Autodesk Fusion 360 part; units mm, degrees
(part 34 of 40)
  line L8870 (236.8217, 91.8506) -> (236.8425, 91.6948) construction
  line L8871 (236.8425, 91.6948) -> (236.8621, 91.5386) construction
  line L8872 (236.8621, 91.5386) -> (236.8805, 91.3821) construction
  line L8873 (236.8805, 91.3821) -> (236.8978, 91.2253) construction
  line L8874 (236.8978, 91.2253) -> (236.9138, 91.0682) construction
  line L8875 (236.9138, 91.0682) -> (236.9285, 90.9107) construction
  line L8876 (236.9285, 90.9107) -> (236.9418, 90.7529) construction
  line L8877 (236.9418, 90.7529) -> (236.9538, 90.5947) construction
  line L8878 (236.9538, 90.5947) -> (236.9645, 90.4362) construction
  line L8879 (236.9645, 90.4362) -> (236.974, 90.2774) construction
  line L8880 (236.974, 90.2774) -> (236.9824, 90.1183) construction
  line L8881 (236.9824, 90.1183) -> (236.9897, 89.9589) construction
  line L8882 (236.9897, 89.9589) -> (236.9958, 89.7993) construction
  line L8883 (236.9958, 89.7993) -> (237.0009, 89.6395) construction
  line L8884 (237.0009, 89.6395) -> (237.0049, 89.4794) construction
  line L8885 (237.0049, 89.4794) -> (237.0077, 89.3191) construction
  line L8886 (237.0077, 89.3191) -> (237.0096, 89.1585) construction
  line L8887 (237.0096, 89.1585) -> (237.0103, 88.9977) construction
  line L8888 (237.0103, 88.9977) -> (237.01, 88.8367) construction
  line L8889 (237.01, 88.8367) -> (237.0086, 88.6755) construction
  line L8890 (237.0086, 88.6755) -> (237.0062, 88.5141) construction
  line L8891 (237.0062, 88.5141) -> (237.0028, 88.3525) construction
  line L8892 (237.0028, 88.3525) -> (236.9985, 88.1907) construction
  line L8893 (236.9985, 88.1907) -> (236.9931, 88.0288) construction
  line L8894 (236.9931, 88.0288) -> (236.9868, 87.8666) construction
  line L8895 (236.9868, 87.8666) -> (236.9795, 87.7043) construction
  line L8896 (236.9795, 87.7043) -> (236.9712, 87.5419) construction
  line L8897 (236.9712, 87.5419) -> (236.962, 87.3793) construction
  line L8898 (236.962, 87.3793) -> (236.9519, 87.2165) construction
  line L8899 (236.9519, 87.2165) -> (236.9408, 87.0536) construction
  line L8900 (236.9408, 87.0536) -> (236.9287, 86.8905) construction
  line L8901 (236.9287, 86.8905) -> (236.9158, 86.7273) construction
  line L8902 (236.9158, 86.7273) -> (236.902, 86.564) construction
  line L8903 (236.902, 86.564) -> (236.8872, 86.4005) construction
  line L8904 (236.8872, 86.4005) -> (236.8716, 86.2369) construction
  line L8905 (236.8716, 86.2369) -> (236.855, 86.0732) construction
  line L8906 (236.855, 86.0732) -> (236.8376, 85.9094) construction
  line L8907 (236.8376, 85.9094) -> (236.8193, 85.7455) construction
  line L8908 (236.8193, 85.7455) -> (236.8001, 85.5815) construction
  line L8909 (236.8001, 85.5815) -> (236.78, 85.4174) construction
  line L8910 (236.78, 85.4174) -> (236.7591, 85.2532) construction
  line L8911 (236.7591, 85.2532) -> (236.7374, 85.0889) construction
  line L8912 (236.7374, 85.0889) -> (236.7148, 84.9245) construction
  line L8913 (236.7148, 84.9245) -> (236.6913, 84.76) construction
  line L8914 (236.6913, 84.76) -> (236.667, 84.5954) construction
  line L8915 (236.667, 84.5954) -> (236.6418, 84.4308) construction
  line L8916 (236.6418, 84.4308) -> (236.6159, 84.266) construction
  line L8917 (236.6159, 84.266) -> (236.5891, 84.1013) construction
  line L8918 (236.5891, 84.1013) -> (236.5614, 83.9364) construction
  line L8919 (236.5614, 83.9364) -> (236.533, 83.7715) construction
  line L8920 (236.533, 83.7715) -> (236.5038, 83.6065) construction
  line L8921 (236.5038, 83.6065) -> (236.4737, 83.4415) construction
  line L8922 (236.4737, 83.4415) -> (236.4428, 83.2764) construction
  line L8923 (236.4428, 83.2764) -> (236.4112, 83.1113) construction
  line L8924 (236.4112, 83.1113) -> (236.3852, 82.9792) construction
  line L8925 (236.3852, 82.9792) -> (236.3654, 82.8801) construction
  line L8926 (236.3654, 82.8801) -> (236.352, 82.814) construction
  line L8927 (236.352, 82.814) -> (236.3452, 82.7809) construction
  arc A219 (171.9828, 209.0993) -> (168.332, 206.4469) centre (212.132, 150) ccw
  arc A220 (181.8522, 201.1066) -> (184.5338, 200.3721) centre (183.5728, 202.1261) ccw
  arc A221 (204.8514, 206.9737) -> (206.5892, 209.1442) centre (204.5979, 208.9575) ccw
  spline S119 degree 5 poles (206.4369, 89.2315) (206.4341, 89.2007) (206.4291, 89.1391) (206.4242, 89.0467) (206.4223, 88.9234) (206.4264, 88.769) (206.4351, 88.6144) (206.4466, 88.4597) (206.4597, 88.305) (206.4737, 88.1502) (206.4889, 87.9955) (206.5055, 87.8407) (206.524, 87.686) (206.5449, 87.5312) (206.5679, 87.3765) (206.593, 87.2218) (206.6199, 87.0671) (206.6482, 86.9125) (206.6778, 86.7579) (206.7087, 86.6034) (206.7407, 86.4489) (206.7741, 86.2945) (206.8088, 86.1402) (206.8449, 85.986) (206.8823, 85.8318) (206.9211, 85.6778) (206.9611, 85.5238) (207.0023, 85.3699) (207.0447, 85.2161) (207.0881, 85.0624) (207.1327, 84.9088) (207.1784, 84.7553) (207.2252, 84.602) (207.2731, 84.4487) (207.3221, 84.2956) (207.3721, 84.1426) (207.4233, 83.9897) (207.4754, 83.8369) (207.5285, 83.6842) (207.5827, 83.5317) (207.6378, 83.3794) (207.694, 83.2271) (207.751, 83.075) (207.8091, 82.923) (207.8681, 82.7712) (207.9281, 82.6196) (207.989, 82.468) (208.0508, 82.3167) (208.1135, 82.1655) (208.1772, 82.0144) (208.2417, 81.8635) (208.3071, 81.7128) (208.3735, 81.5622) (208.4407, 81.4118) (208.5087, 81.2616) (208.5777, 81.1115) (208.6474, 80.9616) (208.7181, 80.8119) (208.7895, 80.6624) (208.8619, 80.513) (208.935, 80.3638) (209.009, 80.2148) (209.0838, 80.066) (209.1594, 79.9174) (209.2358, 79.7689) (209.313, 79.6207) (209.391, 79.4726) (209.4698, 79.3248) (209.5494, 79.1771) (209.6297, 79.0297) (209.7109, 78.8824) (209.7764, 78.7648) (209.8259, 78.6766) (209.8591, 78.6179) (209.8757, 78.5885) knots 0 0 0 0 0 0 0.01428571 0.02857143 0.04285714 0.05714286 0.07142857 0.08571429 0.1 0.11428571 0.12857143 0.14285714 0.15714286 0.17142857 0.18571429 0.2 0.21428571 0.22857143 0.24285714 0.25714286 0.27142857 0.28571429 0.3 0.31428571 0.32857143 0.34285714 0.35714286 0.37142857 0.38571429 0.4 0.41428571 0.42857143 0.44285714 0.45714286 0.47142857 0.48571429 0.5 0.51428571 0.52857143 0.54285714 0.55714286 0.57142857 0.58571429 0.6 0.61428571 0.62857143 0.64285714 0.65714286 0.67142857 0.68571429 0.7 0.71428571 0.72857143 0.74285714 0.75714286 0.77142857 0.78571429 0.8 0.81428571 0.82857143 0.84285714 0.85714286 0.87142857 0.88571429 0.9 0.91428571 0.92857143 0.94285714 0.95714286 0.97142857 0.98571429 1 1 1 1 1 1
  line L8928 (206.4369, 89.2315) -> (206.4341, 89.2007) construction
  line L8929 (206.4341, 89.2007) -> (206.4291, 89.1391) construction
  line L8930 (206.4291, 89.1391) -> (206.4242, 89.0467) construction
  line L8931 (206.4242, 89.0467) -> (206.4223, 88.9234) construction
  line L8932 (206.4223, 88.9234) -> (206.4264, 88.769) construction
  line L8933 (206.4264, 88.769) -> (206.4351, 88.6144) construction
  line L8934 (206.4351, 88.6144) -> (206.4466, 88.4597) construction
  line L8935 (206.4466, 88.4597) -> (206.4597, 88.305) construction
  line L8936 (206.4597, 88.305) -> (206.4737, 88.1502) construction
  line L8937 (206.4737, 88.1502) -> (206.4889, 87.9955) construction
  line L8938 (206.4889, 87.9955) -> (206.5055, 87.8407) construction
  line L8939 (206.5055, 87.8407) -> (206.524, 87.686) construction
  line L8940 (206.524, 87.686) -> (206.5449, 87.5312) construction
  line L8941 (206.5449, 87.5312) -> (206.5679, 87.3765) construction
  line L8942 (206.5679, 87.3765) -> (206.593, 87.2218) construction
  line L8943 (206.593, 87.2218) -> (206.6199, 87.0671) construction
  line L8944 (206.6199, 87.0671) -> (206.6482, 86.9125) construction
  line L8945 (206.6482, 86.9125) -> (206.6778, 86.7579) construction
  line L8946 (206.6778, 86.7579) -> (206.7087, 86.6034) construction
  line L8947 (206.7087, 86.6034) -> (206.7407, 86.4489) construction
  line L8948 (206.7407, 86.4489) -> (206.7741, 86.2945) construction
  line L8949 (206.7741, 86.2945) -> (206.8088, 86.1402) construction
  line L8950 (206.8088, 86.1402) -> (206.8449, 85.986) construction
  line L8951 (206.8449, 85.986) -> (206.8823, 85.8318) construction
  line L8952 (206.8823, 85.8318) -> (206.9211, 85.6778) construction
  line L8953 (206.9211, 85.6778) -> (206.9611, 85.5238) construction
  line L8954 (206.9611, 85.5238) -> (207.0023, 85.3699) construction
  line L8955 (207.0023, 85.3699) -> (207.0447, 85.2161) construction
  line L8956 (207.0447, 85.2161) -> (207.0881, 85.0624) construction
  line L8957 (207.0881, 85.0624) -> (207.1327, 84.9088) construction
  line L8958 (207.1327, 84.9088) -> (207.1784, 84.7553) construction
  line L8959 (207.1784, 84.7553) -> (207.2252, 84.602) construction
  line L8960 (207.2252, 84.602) -> (207.2731, 84.4487) construction
  line L8961 (207.2731, 84.4487) -> (207.3221, 84.2956) construction
  line L8962 (207.3221, 84.2956) -> (207.3721, 84.1426) construction
  line L8963 (207.3721, 84.1426) -> (207.4233, 83.9897) construction
  line L8964 (207.4233, 83.9897) -> (207.4754, 83.8369) construction
  line L8965 (207.4754, 83.8369) -> (207.5285, 83.6842) construction
  line L8966 (207.5285, 83.6842) -> (207.5827, 83.5317) construction
  line L8967 (207.5827, 83.5317) -> (207.6378, 83.3794) construction
  line L8968 (207.6378, 83.3794) -> (207.694, 83.2271) construction
  line L8969 (207.694, 83.2271) -> (207.751, 83.075) construction
  line L8970 (207.751, 83.075) -> (207.8091, 82.923) construction
  line L8971 (207.8091, 82.923) -> (207.8681, 82.7712) construction
  line L8972 (207.8681, 82.7712) -> (207.9281, 82.6196) construction
  line L8973 (207.9281, 82.6196) -> (207.989, 82.468) construction
  line L8974 (207.989, 82.468) -> (208.0508, 82.3167) construction
  line L8975 (208.0508, 82.3167) -> (208.1135, 82.1655) construction
  line L8976 (208.1135, 82.1655) -> (208.1772, 82.0144) construction
  line L8977 (208.1772, 82.0144) -> (208.2417, 81.8635) construction
  line L8978 (208.2417, 81.8635) -> (208.3071, 81.7128) construction
  line L8979 (208.3071, 81.7128) -> (208.3735, 81.5622) construction
  line L8980 (208.3735, 81.5622) -> (208.4407, 81.4118) construction
  line L8981 (208.4407, 81.4118) -> (208.5087, 81.2616) construction
  line L8982 (208.5087, 81.2616) -> (208.5777, 81.1115) construction
  line L8983 (208.5777, 81.1115) -> (208.6474, 80.9616) construction
  line L8984 (208.6474, 80.9616) -> (208.7181, 80.8119) construction
  line L8985 (208.7181, 80.8119) -> (208.7895, 80.6624) construction
  line L8986 (208.7895, 80.6624) -> (208.8619, 80.513) construction
  line L8987 (208.8619, 80.513) -> (208.935, 80.3638) construction
  line L8988 (208.935, 80.3638) -> (209.009, 80.2148) construction
  line L8989 (209.009, 80.2148) -> (209.0838, 80.066) construction
  line L8990 (209.0838, 80.066) -> (209.1594, 79.9174) construction
  line L8991 (209.1594, 79.9174) -> (209.2358, 79.7689) construction
  line L8992 (209.2358, 79.7689) -> (209.313, 79.6207) construction
  line L8993 (209.313, 79.6207) -> (209.391, 79.4726) construction
  line L8994 (209.391, 79.4726) -> (209.4698, 79.3248) construction
  line L8995 (209.4698, 79.3248) -> (209.5494, 79.1771) construction
  line L8996 (209.5494, 79.1771) -> (209.6297, 79.0297) construction
  line L8997 (209.6297, 79.0297) -> (209.7109, 78.8824) construction
  line L8998 (209.7109, 78.8824) -> (209.7764, 78.7648) construction
  line L8999 (209.7764, 78.7648) -> (209.8259, 78.6766) construction
  line L9000 (209.8259, 78.6766) -> (209.8591, 78.6179) construction
  line L9001 (209.8591, 78.6179) -> (209.8757, 78.5885) construction
  arc A222 (279.3511, 125.7868) -> (280.7456, 130.0785) centre (212.132, 150) ccw
  arc A223 (280.7456, 169.9215) -> (279.3511, 174.2132) centre (212.132, 150) ccw
  arc A224 (209.8757, 78.5885) -> (214.3883, 78.5885) centre (212.132, 150) ccw
  arc A225 (283.5435, 147.7437) -> (283.5435, 152.2563) centre (212.132, 150) ccw
  spline S120 degree 5 poles (206.4369, 210.7685) (206.4341, 210.7993) (206.4291, 210.8609) (206.4242, 210.9533) (206.4223, 211.0766) (206.4264, 211.231) (206.4351, 211.3856) (206.4466, 211.5403) (206.4597, 211.695) (206.4737, 211.8498) (206.4889, 212.0045) (206.5055, 212.1593) (206.524, 212.314) (206.5449, 212.4688) (206.5679, 212.6235) (206.593, 212.7782) (206.6199, 212.9329) (206.6482, 213.0875) (206.6778, 213.2421) (206.7087, 213.3966) (206.7407, 213.5511) (206.7741, 213.7055) (206.8088, 213.8598) (206.8449, 214.014) (206.8823, 214.1682) (206.9211, 214.3222) (206.9611, 214.4762) (207.0023, 214.6301) (207.0447, 214.7839) (207.0881, 214.9376) (207.1327, 215.0912) (207.1784, 215.2447) (207.2252, 215.398) (207.2731, 215.5513) (207.3221, 215.7044) (207.3721, 215.8574) (207.4233, 216.0103) (207.4754, 216.1631) (207.5285, 216.3158) (207.5827, 216.4683) (207.6378, 216.6206) (207.694, 216.7729) (207.751, 216.925) (207.8091, 217.077) (207.8681, 217.2288) (207.9281, 217.3804) (207.989, 217.532) (208.0508, 217.6833) (208.1135, 217.8345) (208.1772, 217.9856) (208.2417, 218.1365) (208.3071, 218.2872) (208.3735, 218.4378) (208.4407, 218.5882) (208.5087, 218.7384) (208.5777, 218.8885) (208.6474, 219.0384) (208.7181, 219.1881) (208.7895, 219.3376) (208.8619, 219.487) (208.935, 219.6362) (209.009, 219.7852) (209.0838, 219.934) (209.1594, 220.0826) (209.2358, 220.2311) (209.313, 220.3793) (209.391, 220.5274) (209.4698, 220.6752) (209.5494, 220.8229) (209.6297, 220.9703) (209.7109, 221.1176) (209.7764, 221.2352) (209.8259, 221.3234) (209.8591, 221.3821) (209.8757, 221.4115) knots 0 0 0 0 0 0 0.01428571 0.02857143 0.04285714 0.05714286 0.07142857 0.08571429 0.1 0.11428571 0.12857143 0.14285714 0.15714286 0.17142857 0.18571429 0.2 0.21428571 0.22857143 0.24285714 0.25714286 0.27142857 0.28571429 0.3 0.31428571 0.32857143 0.34285714 0.35714286 0.37142857 0.38571429 0.4 0.41428571 0.42857143 0.44285714 0.45714286 0.47142857 0.48571429 0.5 0.51428571 0.52857143 0.54285714 0.55714286 0.57142857 0.58571429 0.6 0.61428571 0.62857143 0.64285714 0.65714286 0.67142857 0.68571429 0.7 0.71428571 0.72857143 0.74285714 0.75714286 0.77142857 0.78571429 0.8 0.81428571 0.82857143 0.84285714 0.85714286 0.87142857 0.88571429 0.9 0.91428571 0.92857143 0.94285714 0.95714286 0.97142857 0.98571429 1 1 1 1 1 1
  line L9002 (206.4369, 210.7685) -> (206.4341, 210.7993) construction
  line L9003 (206.4341, 210.7993) -> (206.4291, 210.8609) construction
  line L9004 (206.4291, 210.8609) -> (206.4242, 210.9533) construction
  line L9005 (206.4242, 210.9533) -> (206.4223, 211.0766) construction
  line L9006 (206.4223, 211.0766) -> (206.4264, 211.231) construction
  line L9007 (206.4264, 211.231) -> (206.4351, 211.3856) construction
  line L9008 (206.4351, 211.3856) -> (206.4466, 211.5403) construction
  line L9009 (206.4466, 211.5403) -> (206.4597, 211.695) construction
  line L9010 (206.4597, 211.695) -> (206.4737, 211.8498) construction
  line L9011 (206.4737, 211.8498) -> (206.4889, 212.0045) construction
  line L9012 (206.4889, 212.0045) -> (206.5055, 212.1593) construction
  line L9013 (206.5055, 212.1593) -> (206.524, 212.314) construction
  line L9014 (206.524, 212.314) -> (206.5449, 212.4688) construction
  line L9015 (206.5449, 212.4688) -> (206.5679, 212.6235) construction
  line L9016 (206.5679, 212.6235) -> (206.593, 212.7782) construction
  line L9017 (206.593, 212.7782) -> (206.6199, 212.9329) construction
  line L9018 (206.6199, 212.9329) -> (206.6482, 213.0875) construction
  line L9019 (206.6482, 213.0875) -> (206.6778, 213.2421) construction
  line L9020 (206.6778, 213.2421) -> (206.7087, 213.3966) construction
  line L9021 (206.7087, 213.3966) -> (206.7407, 213.5511) construction
  line L9022 (206.7407, 213.5511) -> (206.7741, 213.7055) construction
  line L9023 (206.7741, 213.7055) -> (206.8088, 213.8598) construction
  line L9024 (206.8088, 213.8598) -> (206.8449, 214.014) construction
  line L9025 (206.8449, 214.014) -> (206.8823, 214.1682) construction
  line L9026 (206.8823, 214.1682) -> (206.9211, 214.3222) construction
  line L9027 (206.9211, 214.3222) -> (206.9611, 214.4762) construction
  line L9028 (206.9611, 214.4762) -> (207.0023, 214.6301) construction
  line L9029 (207.0023, 214.6301) -> (207.0447, 214.7839) construction
  line L9030 (207.0447, 214.7839) -> (207.0881, 214.9376) construction
  line L9031 (207.0881, 214.9376) -> (207.1327, 215.0912) construction
  line L9032 (207.1327, 215.0912) -> (207.1784, 215.2447) construction
  line L9033 (207.1784, 215.2447) -> (207.2252, 215.398) construction
  line L9034 (207.2252, 215.398) -> (207.2731, 215.5513) construction
  line L9035 (207.2731, 215.5513) -> (207.3221, 215.7044) construction
  line L9036 (207.3221, 215.7044) -> (207.3721, 215.8574) construction
  line L9037 (207.3721, 215.8574) -> (207.4233, 216.0103) construction
  line L9038 (207.4233, 216.0103) -> (207.4754, 216.1631) construction
  line L9039 (207.4754, 216.1631) -> (207.5285, 216.3158) construction
  line L9040 (207.5285, 216.3158) -> (207.5827, 216.4683) construction
  line L9041 (207.5827, 216.4683) -> (207.6378, 216.6206) construction
  line L9042 (207.6378, 216.6206) -> (207.694, 216.7729) construction
  line L9043 (207.694, 216.7729) -> (207.751, 216.925) construction
  line L9044 (207.751, 216.925) -> (207.8091, 217.077) construction
  line L9045 (207.8091, 217.077) -> (207.8681, 217.2288) construction
  line L9046 (207.8681, 217.2288) -> (207.9281, 217.3804) construction
  line L9047 (207.9281, 217.3804) -> (207.989, 217.532) construction
  line L9048 (207.989, 217.532) -> (208.0508, 217.6833) construction
  line L9049 (208.0508, 217.6833) -> (208.1135, 217.8345) construction
  line L9050 (208.1135, 217.8345) -> (208.1772, 217.9856) construction
  line L9051 (208.1772, 217.9856) -> (208.2417, 218.1365) construction
  line L9052 (208.2417, 218.1365) -> (208.3071, 218.2872) construction
  line L9053 (208.3071, 218.2872) -> (208.3735, 218.4378) construction
  line L9054 (208.3735, 218.4378) -> (208.4407, 218.5882) construction
  line L9055 (208.4407, 218.5882) -> (208.5087, 218.7384) construction
  line L9056 (208.5087, 218.7384) -> (208.5777, 218.8885) construction
  line L9057 (208.5777, 218.8885) -> (208.6474, 219.0384) construction
  line L9058 (208.6474, 219.0384) -> (208.7181, 219.1881) construction
  line L9059 (208.7181, 219.1881) -> (208.7895, 219.3376) construction
  line L9060 (208.7895, 219.3376) -> (208.8619, 219.487) construction
  line L9061 (208.8619, 219.487) -> (208.935, 219.6362) construction
  line L9062 (208.935, 219.6362) -> (209.009, 219.7852) construction
  line L9063 (209.009, 219.7852) -> (209.0838, 219.934) construction
  line L9064 (209.0838, 219.934) -> (209.1594, 220.0826) construction
  line L9065 (209.1594, 220.0826) -> (209.2358, 220.2311) construction
  line L9066 (209.2358, 220.2311) -> (209.313, 220.3793) construction
  line L9067 (209.313, 220.3793) -> (209.391, 220.5274) construction
  line L9068 (209.391, 220.5274) -> (209.4698, 220.6752) construction
  line L9069 (209.4698, 220.6752) -> (209.5494, 220.8229) construction
  line L9070 (209.5494, 220.8229) -> (209.6297, 220.9703) construction
  line L9071 (209.6297, 220.9703) -> (209.7109, 221.1176) construction
  line L9072 (209.7109, 221.1176) -> (209.7764, 221.2352) construction
  line L9073 (209.7764, 221.2352) -> (209.8259, 221.3234) construction
  line L9074 (209.8259, 221.3234) -> (209.8591, 221.3821) construction
  line L9075 (209.8591, 221.3821) -> (209.8757, 221.4115) construction
  arc A226 (252.2812, 90.9007) -> (255.932, 93.5531) centre (212.132, 150) ccw
  arc A227 (268.567, 139.3184) -> (270.0943, 136.995) centre (270.5321, 138.9465) ccw
  arc A228 (214.3883, 221.4115) -> (209.8757, 221.4115) centre (212.132, 150) ccw
  spline S121 degree 5 poles (156.0975, 125.8052) (156.0692, 125.7929) (156.0122, 125.7692) (155.9258, 125.736) (155.8091, 125.6961) (155.6609, 125.6522) (155.5112, 125.6127) (155.3606, 125.5759) (155.2094, 125.5405) (155.0579, 125.506) (154.906, 125.4726) (154.7537, 125.4406) (154.6008, 125.4104) (154.4472, 125.3824) (154.2929, 125.3565) (154.138, 125.3326) (153.9826, 125.3103) (153.8268, 125.2895) (153.6706, 125.2699) (153.5141, 125.2515) (153.3573, 125.2342) (153.2002, 125.2182) (153.0427, 125.2035) (152.8849, 125.1902) (152.7267, 125.1782) (152.5682, 125.1675) (152.4094, 125.158) (152.2503, 125.1496) (152.0909, 125.1423) (151.9313, 125.1362) (151.7715, 125.1311) (151.6114, 125.1271) (151.4511, 125.1243) (151.2905, 125.1224) (151.1297, 125.1217) (150.9687, 125.122) (150.8075, 125.1234) (150.6461, 125.1258) (150.4845, 125.1292) (150.3227, 125.1335) (150.1608, 125.1389) (149.9986, 125.1452) (149.8363, 125.1525) (149.6739, 125.1608) (149.5113, 125.17) (149.3485, 125.1801) (149.1856, 125.1912) (149.0225, 125.2033) (148.8593, 125.2162) (148.696, 125.23) (148.5325, 125.2448) (148.3689, 125.2604) (148.2052, 125.277) (148.0414, 125.2944) (147.8775, 125.3127) (147.7135, 125.3319) (147.5494, 125.352) (147.3852, 125.3729) (147.2209, 125.3946) (147.0565, 125.4172) (146.892, 125.4407) (146.7274, 125.465) (146.5628, 125.4902) (146.398, 125.5161) (146.2333, 125.5429) (146.0684, 125.5706) (145.9035, 125.599) (145.7385, 125.6282) (145.5735, 125.6583) (145.4084, 125.6892) (145.2433, 125.7208) (145.1112, 125.7468) (145.0121, 125.7666) (144.946, 125.78) (144.9129, 125.7868) knots 0 0 0 0 0 0 0.01428571 0.02857143 0.04285714 0.05714286 0.07142857 0.08571429 0.1 0.11428571 0.12857143 0.14285714 0.15714286 0.17142857 0.18571429 0.2 0.21428571 0.22857143 0.24285714 0.25714286 0.27142857 0.28571429 0.3 0.31428571 0.32857143 0.34285714 0.35714286 0.37142857 0.38571429 0.4 0.41428571 0.42857143 0.44285714 0.45714286 0.47142857 0.48571429 0.5 0.51428571 0.52857143 0.54285714 0.55714286 0.57142857 0.58571429 0.6 0.61428571 0.62857143 0.64285714 0.65714286 0.67142857 0.68571429 0.7 0.71428571 0.72857143 0.74285714 0.75714286 0.77142857 0.78571429 0.8 0.81428571 0.82857143 0.84285714 0.85714286 0.87142857 0.88571429 0.9 0.91428571 0.92857143 0.94285714 0.95714286 0.97142857 0.98571429 1 1 1 1 1 1
  line L9076 (156.0975, 125.8052) -> (156.0692, 125.7929) construction
  line L9077 (156.0692, 125.7929) -> (156.0122, 125.7692) construction
  line L9078 (156.0122, 125.7692) -> (155.9258, 125.736) construction
  line L9079 (155.9258, 125.736) -> (155.8091, 125.6961) construction
  line L9080 (155.8091, 125.6961) -> (155.6609, 125.6522) construction
  line L9081 (155.6609, 125.6522) -> (155.5112, 125.6127) construction
  line L9082 (155.5112, 125.6127) -> (155.3606, 125.5759) construction
  line L9083 (155.3606, 125.5759) -> (155.2094, 125.5405) construction
  line L9084 (155.2094, 125.5405) -> (155.0579, 125.506) construction
  line L9085 (155.0579, 125.506) -> (154.906, 125.4726) construction
  line L9086 (154.906, 125.4726) -> (154.7537, 125.4406) construction
  line L9087 (154.7537, 125.4406) -> (154.6008, 125.4104) construction
  line L9088 (154.6008, 125.4104) -> (154.4472, 125.3824) construction
  line L9089 (154.4472, 125.3824) -> (154.2929, 125.3565) construction
  line L9090 (154.2929, 125.3565) -> (154.138, 125.3326) construction
  line L9091 (154.138, 125.3326) -> (153.9826, 125.3103) construction
  line L9092 (153.9826, 125.3103) -> (153.8268, 125.2895) construction
  line L9093 (153.8268, 125.2895) -> (153.6706, 125.2699) construction
  line L9094 (153.6706, 125.2699) -> (153.5141, 125.2515) construction
  line L9095 (153.5141, 125.2515) -> (153.3573, 125.2342) construction
  line L9096 (153.3573, 125.2342) -> (153.2002, 125.2182) construction
  line L9097 (153.2002, 125.2182) -> (153.0427, 125.2035) construction
  line L9098 (153.0427, 125.2035) -> (152.8849, 125.1902) construction
  line L9099 (152.8849, 125.1902) -> (152.7267, 125.1782) construction
  line L9100 (152.7267, 125.1782) -> (152.5682, 125.1675) construction
  line L9101 (152.5682, 125.1675) -> (152.4094, 125.158) construction
  line L9102 (152.4094, 125.158) -> (152.2503, 125.1496) construction
  line L9103 (152.2503, 125.1496) -> (152.0909, 125.1423) construction
  line L9104 (152.0909, 125.1423) -> (151.9313, 125.1362) construction
  line L9105 (151.9313, 125.1362) -> (151.7715, 125.1311) construction
  line L9106 (151.7715, 125.1311) -> (151.6114, 125.1271) construction
  line L9107 (151.6114, 125.1271) -> (151.4511, 125.1243) construction
  line L9108 (151.4511, 125.1243) -> (151.2905, 125.1224) construction
  line L9109 (151.2905, 125.1224) -> (151.1297, 125.1217) construction
  line L9110 (151.1297, 125.1217) -> (150.9687, 125.122) construction
  line L9111 (150.9687, 125.122) -> (150.8075, 125.1234) construction
  line L9112 (150.8075, 125.1234) -> (150.6461, 125.1258) construction
  line L9113 (150.6461, 125.1258) -> (150.4845, 125.1292) construction
  line L9114 (150.4845, 125.1292) -> (150.3227, 125.1335) construction
  line L9115 (150.3227, 125.1335) -> (150.1608, 125.1389) construction
  line L9116 (150.1608, 125.1389) -> (149.9986, 125.1452) construction
  line L9117 (149.9986, 125.1452) -> (149.8363, 125.1525) construction
  line L9118 (149.8363, 125.1525) -> (149.6739, 125.1608) construction
  line L9119 (149.6739, 125.1608) -> (149.5113, 125.17) construction
  line L9120 (149.5113, 125.17) -> (149.3485, 125.1801) construction
  line L9121 (149.3485, 125.1801) -> (149.1856, 125.1912) construction
  line L9122 (149.1856, 125.1912) -> (149.0225, 125.2033) construction
  line L9123 (149.0225, 125.2033) -> (148.8593, 125.2162) construction
  line L9124 (148.8593, 125.2162) -> (148.696, 125.23) construction
  line L9125 (148.696, 125.23) -> (148.5325, 125.2448) construction
  line L9126 (148.5325, 125.2448) -> (148.3689, 125.2604) construction
  line L9127 (148.3689, 125.2604) -> (148.2052, 125.277) construction
  line L9128 (148.2052, 125.277) -> (148.0414, 125.2944) construction
  line L9129 (148.0414, 125.2944) -> (147.8775, 125.3127) construction
  line L9130 (147.8775, 125.3127) -> (147.7135, 125.3319) construction
  line L9131 (147.7135, 125.3319) -> (147.5494, 125.352) construction
  line L9132 (147.5494, 125.352) -> (147.3852, 125.3729) construction
  line L9133 (147.3852, 125.3729) -> (147.2209, 125.3946) construction
  line L9134 (147.2209, 125.3946) -> (147.0565, 125.4172) construction
  line L9135 (147.0565, 125.4172) -> (146.892, 125.4407) construction
  line L9136 (146.892, 125.4407) -> (146.7274, 125.465) construction
  line L9137 (146.7274, 125.465) -> (146.5628, 125.4902) construction
  line L9138 (146.5628, 125.4902) -> (146.398, 125.5161) construction
  line L9139 (146.398, 125.5161) -> (146.2333, 125.5429) construction
  line L9140 (146.2333, 125.5429) -> (146.0684, 125.5706) construction
  line L9141 (146.0684, 125.5706) -> (145.9035, 125.599) construction
  line L9142 (145.9035, 125.599) -> (145.7385, 125.6282) construction
  line L9143 (145.7385, 125.6282) -> (145.5735, 125.6583) construction
  line L9144 (145.5735, 125.6583) -> (145.4084, 125.6892) construction
  line L9145 (145.4084, 125.6892) -> (145.2433, 125.7208) construction
  line L9146 (145.2433, 125.7208) -> (145.1112, 125.7468) construction
  line L9147 (145.1112, 125.7468) -> (145.0121, 125.7666) construction
  line L9148 (145.0121, 125.7666) -> (144.946, 125.78) construction
  line L9149 (144.946, 125.78) -> (144.9129, 125.7868) construction
  arc A229 (222.8136, 206.435) -> (225.137, 207.9623) centre (223.1855, 208.4001) ccw
  arc A230 (170.3188, 110.6216) -> (167.5414, 110.7517) centre (168.8628, 109.2504) ccw
  arc A231 (161.7599, 177.5982) -> (161.0254, 180.2798) centre (160.0059, 178.5592) ccw
  arc A232 (201.4504, 93.565) -> (199.127, 92.0377) centre (201.0785, 91.5999) ccw
  arc A233 (188.5839, 95.4634) -> (187.6019, 98.0646) centre (186.7478, 96.2562) ccw
  line L9150 (157.5954, 126.4519) -> (156.0975, 125.8052)
  line L9151 (270.0943, 163.005) -> (271.6862, 163.3622)
  arc A234 (235.6801, 204.5366) -> (236.6621, 201.9354) centre (237.5162, 203.7438) ccw
  line L9152 (271.2762, 144.4572) -> (272.9005, 144.3049)
  line L9153 (266.6686, 126.4519) -> (268.1665, 125.8052)
  arc A235 (181.8522, 201.1066) -> (184.5338, 200.3721) centre (183.5728, 202.1261) ccw
  arc A236 (161.0254, 119.7202) -> (161.7599, 122.4018) centre (160.0059, 121.4408) ccw
  arc A237 (155.697, 160.6816) -> (154.1697, 163.005) centre (153.7319, 161.0535) ccw
  spline S122 degree 5 poles (257.9473, 190.3263) (257.9705, 190.3467) (258.0174, 190.3868) (258.0893, 190.4451) (258.188, 190.5192) (258.3153, 190.6066) (258.4455, 190.6904) (258.5774, 190.772) (258.7102, 190.8524) (258.8437, 190.932) (258.9778, 191.0107) (259.1127, 191.0883) (259.2488, 191.1642) (259.3863, 191.2383) (259.525, 191.3106) (259.6649, 191.3813) (259.8058, 191.4504) (259.9476, 191.5184) (260.0901, 191.5853) (260.2332, 191.6512) (260.377, 191.716) (260.5215, 191.7798) (260.6667, 191.8424) (260.8127, 191.9039) (260.9594, 191.9642) (261.1069, 192.0234) (261.255, 192.0815) (261.4037, 192.1386) (261.553, 192.1947) (261.7029, 192.2499) (261.8534, 192.3041) (262.0044, 192.3574) (262.156, 192.4097) (262.3081, 192.461) (262.4608, 192.5114) (262.614, 192.5608) (262.7678, 192.6094) (262.922, 192.657) (263.0767, 192.7037) (263.2319, 192.7495) (263.3876, 192.7945) (263.5438, 192.8386) (263.7004, 192.8818) (263.8575, 192.9241) (264.015, 192.9656) (264.1729, 193.0063) (264.3313, 193.0461) (264.4901, 193.085) (264.6493, 193.1231) (264.8089, 193.1604) (264.9689, 193.1969) (265.1293, 193.2326) (265.2901, 193.2674) (265.4513, 193.3015) (265.6129, 193.3347) (265.7748, 193.3672) (265.9371, 193.3988) (266.0997, 193.4297) (266.2627, 193.4597) (266.426, 193.489) (266.5897, 193.5175) (266.7537, 193.5453) (266.9181, 193.5723) (267.0828, 193.5984) (267.2478, 193.6239) (267.4131, 193.6486) (267.5787, 193.6725) (267.7446, 193.6956) (267.9109, 193.718) (268.0774, 193.7397) (268.2442, 193.7606) (268.3779, 193.7767) (268.4783, 193.7885) (268.5453, 193.7962) (268.5789, 193.8) knots 0 0 0 0 0 0 0.01428571 0.02857143 0.04285714 0.05714286 0.07142857 0.08571429 0.1 0.11428571 0.12857143 0.14285714 0.15714286 0.17142857 0.18571429 0.2 0.21428571 0.22857143 0.24285714 0.25714286 0.27142857 0.28571429 0.3 0.31428571 0.32857143 0.34285714 0.35714286 0.37142857 0.38571429 0.4 0.41428571 0.42857143 0.44285714 0.45714286 0.47142857 0.48571429 0.5 0.51428571 0.52857143 0.54285714 0.55714286 0.57142857 0.58571429 0.6 0.61428571 0.62857143 0.64285714 0.65714286 0.67142857 0.68571429 0.7 0.71428571 0.72857143 0.74285714 0.75714286 0.77142857 0.78571429 0.8 0.81428571 0.82857143 0.84285714 0.85714286 0.87142857 0.88571429 0.9 0.91428571 0.92857143 0.94285714 0.95714286 0.97142857 0.98571429 1 1 1 1 1 1
  line L9154 (257.9473, 190.3263) -> (257.9705, 190.3467) construction
  line L9155 (257.9705, 190.3467) -> (258.0174, 190.3868) construction
  line L9156 (258.0174, 190.3868) -> (258.0893, 190.4451) construction
  line L9157 (258.0893, 190.4451) -> (258.188, 190.5192) construction
  line L9158 (258.188, 190.5192) -> (258.3153, 190.6066) construction
  line L9159 (258.3153, 190.6066) -> (258.4455, 190.6904) construction
  line L9160 (258.4455, 190.6904) -> (258.5774, 190.772) construction
  line L9161 (258.5774, 190.772) -> (258.7102, 190.8524) construction
  line L9162 (258.7102, 190.8524) -> (258.8437, 190.932) construction
  line L9163 (258.8437, 190.932) -> (258.9778, 191.0107) construction
  line L9164 (258.9778, 191.0107) -> (259.1127, 191.0883) construction
  line L9165 (259.1127, 191.0883) -> (259.2488, 191.1642) construction
  line L9166 (259.2488, 191.1642) -> (259.3863, 191.2383) construction
  line L9167 (259.3863, 191.2383) -> (259.525, 191.3106) construction
  line L9168 (259.525, 191.3106) -> (259.6649, 191.3813) construction
  line L9169 (259.6649, 191.3813) -> (259.8058, 191.4504) construction
  line L9170 (259.8058, 191.4504) -> (259.9476, 191.5184) construction
  line L9171 (259.9476, 191.5184) -> (260.0901, 191.5853) construction
  line L9172 (260.0901, 191.5853) -> (260.2332, 191.6512) construction
  line L9173 (260.2332, 191.6512) -> (260.377, 191.716) construction
  line L9174 (260.377, 191.716) -> (260.5215, 191.7798) construction
  line L9175 (260.5215, 191.7798) -> (260.6667, 191.8424) construction
  line L9176 (260.6667, 191.8424) -> (260.8127, 191.9039) construction
  line L9177 (260.8127, 191.9039) -> (260.9594, 191.9642) construction
  line L9178 (260.9594, 191.9642) -> (261.1069, 192.0234) construction
  line L9179 (261.1069, 192.0234) -> (261.255, 192.0815) construction
  line L9180 (261.255, 192.0815) -> (261.4037, 192.1386) construction
  line L9181 (261.4037, 192.1386) -> (261.553, 192.1947) construction
  line L9182 (261.553, 192.1947) -> (261.7029, 192.2499) construction
  line L9183 (261.7029, 192.2499) -> (261.8534, 192.3041) construction
  line L9184 (261.8534, 192.3041) -> (262.0044, 192.3574) construction
  line L9185 (262.0044, 192.3574) -> (262.156, 192.4097) construction
  line L9186 (262.156, 192.4097) -> (262.3081, 192.461) construction
  line L9187 (262.3081, 192.461) -> (262.4608, 192.5114) construction
  line L9188 (262.4608, 192.5114) -> (262.614, 192.5608) construction
  line L9189 (262.614, 192.5608) -> (262.7678, 192.6094) construction
  line L9190 (262.7678, 192.6094) -> (262.922, 192.657) construction
  line L9191 (262.922, 192.657) -> (263.0767, 192.7037) construction
  line L9192 (263.0767, 192.7037) -> (263.2319, 192.7495) construction
  line L9193 (263.2319, 192.7495) -> (263.3876, 192.7945) construction
  line L9194 (263.3876, 192.7945) -> (263.5438, 192.8386) construction
  line L9195 (263.5438, 192.8386) -> (263.7004, 192.8818) construction
  line L9196 (263.7004, 192.8818) -> (263.8575, 192.9241) construction
  line L9197 (263.8575, 192.9241) -> (264.015, 192.9656) construction
  line L9198 (264.015, 192.9656) -> (264.1729, 193.0063) construction
  line L9199 (264.1729, 193.0063) -> (264.3313, 193.0461) construction
  line L9200 (264.3313, 193.0461) -> (264.4901, 193.085) construction
  line L9201 (264.4901, 193.085) -> (264.6493, 193.1231) construction
  line L9202 (264.6493, 193.1231) -> (264.8089, 193.1604) construction
  line L9203 (264.8089, 193.1604) -> (264.9689, 193.1969) construction
  line L9204 (264.9689, 193.1969) -> (265.1293, 193.2326) construction
  line L9205 (265.1293, 193.2326) -> (265.2901, 193.2674) construction
  line L9206 (265.2901, 193.2674) -> (265.4513, 193.3015) construction
  line L9207 (265.4513, 193.3015) -> (265.6129, 193.3347) construction
  line L9208 (265.6129, 193.3347) -> (265.7748, 193.3672) construction
  line L9209 (265.7748, 193.3672) -> (265.9371, 193.3988) construction
  line L9210 (265.9371, 193.3988) -> (266.0997, 193.4297) construction
  line L9211 (266.0997, 193.4297) -> (266.2627, 193.4597) construction
  line L9212 (266.2627, 193.4597) -> (266.426, 193.489) construction
  line L9213 (266.426, 193.489) -> (266.5897, 193.5175) construction
  line L9214 (266.5897, 193.5175) -> (266.7537, 193.5453) construction
  line L9215 (266.7537, 193.5453) -> (266.9181, 193.5723) construction
  line L9216 (266.9181, 193.5723) -> (267.0828, 193.5984) construction
  line L9217 (267.0828, 193.5984) -> (267.2478, 193.6239) construction
  line L9218 (267.2478, 193.6239) -> (267.4131, 193.6486) construction
  line L9219 (267.4131, 193.6486) -> (267.5787, 193.6725) construction
  line L9220 (267.5787, 193.6725) -> (267.7446, 193.6956) construction
  line L9221 (267.7446, 193.6956) -> (267.9109, 193.718) construction
  line L9222 (267.9109, 193.718) -> (268.0774, 193.7397) construction
  line L9223 (268.0774, 193.7397) -> (268.2442, 193.7606) construction
  line L9224 (268.2442, 193.7606) -> (268.3779, 193.7767) construction
  line L9225 (268.3779, 193.7767) -> (268.4783, 193.7885) construction
  line L9226 (268.4783, 193.7885) -> (268.5453, 193.7962) construction
  line L9227 (268.5453, 193.7962) -> (268.5789, 193.8) construction
  spline S123 degree 5 poles (159.6217, 181.1115) (159.5952, 181.1272) (159.5425, 181.1594) (159.4648, 181.2097) (159.3639, 181.2807) (159.2414, 181.3748) (159.1214, 181.4727) (159.0031, 181.5729) (158.8856, 181.6744) (158.7686, 181.7767) (158.6523, 181.88) (158.5369, 181.9844) (158.4226, 182.0903) (158.3096, 182.1981) (158.198, 182.3077) (158.0876, 182.419) (157.9783, 182.5316) (157.8698, 182.6455) (157.7622, 182.7603) (157.6553, 182.876) (157.5492, 182.9927) (157.4439, 183.1105) (157.3394, 183.2292) (157.2359, 183.3491) (157.1332, 183.47) (157.0313, 183.5919) (156.9303, 183.7148) (156.83, 183.8386) (156.7305, 183.9633) (156.6317, 184.0888) (156.5336, 184.2151) (156.4363, 184.3423) (156.3397, 184.4703) (156.2439, 184.5991) (156.1488, 184.7288) (156.0544, 184.8592) (155.9608, 184.9905) (155.8678, 185.1224) (155.7756, 185.2552) (155.684, 185.3886) (155.5932, 185.5228) (155.503, 185.6577) (155.4135, 185.7933) (155.3247, 185.9295) (155.2365, 186.0665) (155.1491, 186.2042) (155.0623, 186.3425) (154.9762, 186.4815) (154.8907, 186.6211) (154.8059, 186.7614) (154.7218, 186.9023) (154.6383, 187.0438) (154.5555, 187.186) (154.4733, 187.3288) (154.3917, 187.4721) (154.3108, 187.6161) (154.2306, 187.7607) (154.151, 187.9058) (154.072, 188.0515) (153.9937, 188.1978) (153.916, 188.3447) (153.8389, 188.4921) (153.7625, 188.6401) (153.6867, 188.7886) (153.6115, 188.9377) (153.537, 189.0873) (153.463, 189.2374) (153.3897, 189.3881) (153.3171, 189.5393) (153.245, 189.6909) (153.1736, 189.8431) (153.1169, 189.9653) (153.0747, 190.0572) (153.0467, 190.1185) (153.0327, 190.1492) knots 0 0 0 0 0 0 0.01428571 0.02857143 0.04285714 0.05714286 0.07142857 0.08571429 0.1 0.11428571 0.12857143 0.14285714 0.15714286 0.17142857 0.18571429 0.2 0.21428571 0.22857143 0.24285714 0.25714286 0.27142857 0.28571429 0.3 0.31428571 0.32857143 0.34285714 0.35714286 0.37142857 0.38571429 0.4 0.41428571 0.42857143 0.44285714 0.45714286 0.47142857 0.48571429 0.5 0.51428571 0.52857143 0.54285714 0.55714286 0.57142857 0.58571429 0.6 0.61428571 0.62857143 0.64285714 0.65714286 0.67142857 0.68571429 0.7 0.71428571 0.72857143 0.74285714 0.75714286 0.77142857 0.78571429 0.8 0.81428571 0.82857143 0.84285714 0.85714286 0.87142857 0.88571429 0.9 0.91428571 0.92857143 0.94285714 0.95714286 0.97142857 0.98571429 1 1 1 1 1 1
  line L9228 (159.6217, 181.1115) -> (159.5952, 181.1272) construction
  line L9229 (159.5952, 181.1272) -> (159.5425, 181.1594) construction
  line L9230 (159.5425, 181.1594) -> (159.4648, 181.2097) construction
  line L9231 (159.4648, 181.2097) -> (159.3639, 181.2807) construction
  line L9232 (159.3639, 181.2807) -> (159.2414, 181.3748) construction
  line L9233 (159.2414, 181.3748) -> (159.1214, 181.4727) construction
  line L9234 (159.1214, 181.4727) -> (159.0031, 181.5729) construction
  line L9235 (159.0031, 181.5729) -> (158.8856, 181.6744) construction
  line L9236 (158.8856, 181.6744) -> (158.7686, 181.7767) construction
  line L9237 (158.7686, 181.7767) -> (158.6523, 181.88) construction
  line L9238 (158.6523, 181.88) -> (158.5369, 181.9844) construction
  line L9239 (158.5369, 181.9844) -> (158.4226, 182.0903) construction
  line L9240 (158.4226, 182.0903) -> (158.3096, 182.1981) construction
  line L9241 (158.3096, 182.1981) -> (158.198, 182.3077) construction
  line L9242 (158.198, 182.3077) -> (158.0876, 182.419) construction
  line L9243 (158.0876, 182.419) -> (157.9783, 182.5316) construction
  line L9244 (157.9783, 182.5316) -> (157.8698, 182.6455) construction
  line L9245 (157.8698, 182.6455) -> (157.7622, 182.7603) construction
  line L9246 (157.7622, 182.7603) -> (157.6553, 182.876) construction
  line L9247 (157.6553, 182.876) -> (157.5492, 182.9927) construction
  line L9248 (157.5492, 182.9927) -> (157.4439, 183.1105) construction
  line L9249 (157.4439, 183.1105) -> (157.3394, 183.2292) construction
  line L9250 (157.3394, 183.2292) -> (157.2359, 183.3491) construction
  line L9251 (157.2359, 183.3491) -> (157.1332, 183.47) construction
  line L9252 (157.1332, 183.47) -> (157.0313, 183.5919) construction
  line L9253 (157.0313, 183.5919) -> (156.9303, 183.7148) construction
  line L9254 (156.9303, 183.7148) -> (156.83, 183.8386) construction
  line L9255 (156.83, 183.8386) -> (156.7305, 183.9633) construction
  line L9256 (156.7305, 183.9633) -> (156.6317, 184.0888) construction
  line L9257 (156.6317, 184.0888) -> (156.5336, 184.2151) construction
  line L9258 (156.5336, 184.2151) -> (156.4363, 184.3423) construction
  line L9259 (156.4363, 184.3423) -> (156.3397, 184.4703) construction
  line L9260 (156.3397, 184.4703) -> (156.2439, 184.5991) construction
  line L9261 (156.2439, 184.5991) -> (156.1488, 184.7288) construction
  line L9262 (156.1488, 184.7288) -> (156.0544, 184.8592) construction
  line L9263 (156.0544, 184.8592) -> (155.9608, 184.9905) construction
  line L9264 (155.9608, 184.9905) -> (155.8678, 185.1224) construction
  line L9265 (155.8678, 185.1224) -> (155.7756, 185.2552) construction
  line L9266 (155.7756, 185.2552) -> (155.684, 185.3886) construction
  line L9267 (155.684, 185.3886) -> (155.5932, 185.5228) construction
  line L9268 (155.5932, 185.5228) -> (155.503, 185.6577) construction
  line L9269 (155.503, 185.6577) -> (155.4135, 185.7933) construction
  line L9270 (155.4135, 185.7933) -> (155.3247, 185.9295) construction
  line L9271 (155.3247, 185.9295) -> (155.2365, 186.0665) construction
  line L9272 (155.2365, 186.0665) -> (155.1491, 186.2042) construction
  line L9273 (155.1491, 186.2042) -> (155.0623, 186.3425) construction
  line L9274 (155.0623, 186.3425) -> (154.9762, 186.4815) construction
  line L9275 (154.9762, 186.4815) -> (154.8907, 186.6211) construction
  line L9276 (154.8907, 186.6211) -> (154.8059, 186.7614) construction
  line L9277 (154.8059, 186.7614) -> (154.7218, 186.9023) construction
  line L9278 (154.7218, 186.9023) -> (154.6383, 187.0438) construction
  line L9279 (154.6383, 187.0438) -> (154.5555, 187.186) construction
  line L9280 (154.5555, 187.186) -> (154.4733, 187.3288) construction
  line L9281 (154.4733, 187.3288) -> (154.3917, 187.4721) construction
  line L9282 (154.3917, 187.4721) -> (154.3108, 187.6161) construction
  line L9283 (154.3108, 187.6161) -> (154.2306, 187.7607) construction
  line L9284 (154.2306, 187.7607) -> (154.151, 187.9058) construction
  line L9285 (154.151, 187.9058) -> (154.072, 188.0515) construction
  line L9286 (154.072, 188.0515) -> (153.9937, 188.1978) construction
  line L9287 (153.9937, 188.1978) -> (153.916, 188.3447) construction
  line L9288 (153.916, 188.3447) -> (153.8389, 188.4921) construction
  line L9289 (153.8389, 188.4921) -> (153.7625, 188.6401) construction
  line L9290 (153.7625, 188.6401) -> (153.6867, 188.7886) construction
  line L9291 (153.6867, 188.7886) -> (153.6115, 188.9377) construction
  line L9292 (153.6115, 188.9377) -> (153.537, 189.0873) construction
  line L9293 (153.537, 189.0873) -> (153.463, 189.2374) construction
  line L9294 (153.463, 189.2374) -> (153.3897, 189.3881) construction
  line L9295 (153.3897, 189.3881) -> (153.3171, 189.5393) construction
  line L9296 (153.3171, 189.5393) -> (153.245, 189.6909) construction
  line L9297 (153.245, 189.6909) -> (153.1736, 189.8431) construction
  line L9298 (153.1736, 189.8431) -> (153.1169, 189.9653) construction
  line L9299 (153.1169, 189.9653) -> (153.0747, 190.0572) construction
  line L9300 (153.0747, 190.0572) -> (153.0467, 190.1185) construction
  line L9301 (153.0467, 190.1185) -> (153.0327, 190.1492) construction
  spline S124 degree 5 poles (268.1665, 125.8052) (268.1948, 125.7929) (268.2518, 125.7692) (268.3382, 125.736) (268.4549, 125.6961) (268.6031, 125.6522) (268.7528, 125.6127) (268.9034, 125.5759) (269.0546, 125.5405) (269.2061, 125.506) (269.358, 125.4726) (269.5103, 125.4406) (269.6632, 125.4104) (269.8168, 125.3824) (269.9711, 125.3565) (270.126, 125.3326) (270.2814, 125.3103) (270.4372, 125.2895) (270.5934, 125.2699) (270.7499, 125.2515) (270.9067, 125.2342) (271.0638, 125.2182) (271.2213, 125.2035) (271.3791, 125.1902) (271.5373, 125.1782) (271.6958, 125.1675) (271.8546, 125.158) (272.0137, 125.1496) (272.1731, 125.1423) (272.3327, 125.1362) (272.4925, 125.1311) (272.6526, 125.1271) (272.8129, 125.1243) (272.9735, 125.1224) (273.1343, 125.1217) (273.2953, 125.122) (273.4565, 125.1234) (273.6179, 125.1258) (273.7795, 125.1292) (273.9413, 125.1335) (274.1032, 125.1389) (274.2654, 125.1452) (274.4277, 125.1525) (274.5901, 125.1608) (274.7527, 125.17) (274.9155, 125.1801) (275.0784, 125.1912) (275.2415, 125.2033) (275.4047, 125.2162) (275.568, 125.23) (275.7315, 125.2448) (275.8951, 125.2604) (276.0588, 125.277) (276.2226, 125.2944) (276.3865, 125.3127) (276.5505, 125.3319) (276.7146, 125.352) (276.8788, 125.3729) (277.0431, 125.3946) (277.2075, 125.4172) (277.372, 125.4407) (277.5366, 125.465) (277.7012, 125.4902) (277.866, 125.5161) (278.0307, 125.5429) (278.1956, 125.5706) (278.3605, 125.599) (278.5255, 125.6282) (278.6905, 125.6583) (278.8556, 125.6892) (279.0207, 125.7208) (279.1528, 125.7468) (279.2519, 125.7666) (279.318, 125.78) (279.3511, 125.7868) knots 0 0 0 0 0 0 0.01428571 0.02857143 0.04285714 0.05714286 0.07142857 0.08571429 0.1 0.11428571 0.12857143 0.14285714 0.15714286 0.17142857 0.18571429 0.2 0.21428571 0.22857143 0.24285714 0.25714286 0.27142857 0.28571429 0.3 0.31428571 0.32857143 0.34285714 0.35714286 0.37142857 0.38571429 0.4 0.41428571 0.42857143 0.44285714 0.45714286 0.47142857 0.48571429 0.5 0.51428571 0.52857143 0.54285714 0.55714286 0.57142857 0.58571429 0.6 0.61428571 0.62857143 0.64285714 0.65714286 0.67142857 0.68571429 0.7 0.71428571 0.72857143 0.74285714 0.75714286 0.77142857 0.78571429 0.8 0.81428571 0.82857143 0.84285714 0.85714286 0.87142857 0.88571429 0.9 0.91428571 0.92857143 0.94285714 0.95714286 0.97142857 0.98571429 1 1 1 1 1 1
  line L9302 (268.1665, 125.8052) -> (268.1948, 125.7929) construction
  line L9303 (268.1948, 125.7929) -> (268.2518, 125.7692) construction
  line L9304 (268.2518, 125.7692) -> (268.3382, 125.736) construction
  line L9305 (268.3382, 125.736) -> (268.4549, 125.6961) construction
  line L9306 (268.4549, 125.6961) -> (268.6031, 125.6522) construction
  line L9307 (268.6031, 125.6522) -> (268.7528, 125.6127) construction
  line L9308 (268.7528, 125.6127) -> (268.9034, 125.5759) construction
  line L9309 (268.9034, 125.5759) -> (269.0546, 125.5405) construction
  line L9310 (269.0546, 125.5405) -> (269.2061, 125.506) construction
  line L9311 (269.2061, 125.506) -> (269.358, 125.4726) construction
  line L9312 (269.358, 125.4726) -> (269.5103, 125.4406) construction
  line L9313 (269.5103, 125.4406) -> (269.6632, 125.4104) construction
  line L9314 (269.6632, 125.4104) -> (269.8168, 125.3824) construction
  line L9315 (269.8168, 125.3824) -> (269.9711, 125.3565) construction
  line L9316 (269.9711, 125.3565) -> (270.126, 125.3326) construction
  line L9317 (270.126, 125.3326) -> (270.2814, 125.3103) construction
  line L9318 (270.2814, 125.3103) -> (270.4372, 125.2895) construction
  line L9319 (270.4372, 125.2895) -> (270.5934, 125.2699) construction
  line L9320 (270.5934, 125.2699) -> (270.7499, 125.2515) construction
  line L9321 (270.7499, 125.2515) -> (270.9067, 125.2342) construction
  line L9322 (270.9067, 125.2342) -> (271.0638, 125.2182) construction
  line L9323 (271.0638, 125.2182) -> (271.2213, 125.2035) construction
  line L9324 (271.2213, 125.2035) -> (271.3791, 125.1902) construction
  line L9325 (271.3791, 125.1902) -> (271.5373, 125.1782) construction
  line L9326 (271.5373, 125.1782) -> (271.6958, 125.1675) construction
  line L9327 (271.6958, 125.1675) -> (271.8546, 125.158) construction
  line L9328 (271.8546, 125.158) -> (272.0137, 125.1496) construction
  line L9329 (272.0137, 125.1496) -> (272.1731, 125.1423) construction
  line L9330 (272.1731, 125.1423) -> (272.3327, 125.1362) construction
  line L9331 (272.3327, 125.1362) -> (272.4925, 125.1311) construction
  line L9332 (272.4925, 125.1311) -> (272.6526, 125.1271) construction
  line L9333 (272.6526, 125.1271) -> (272.8129, 125.1243) construction
  line L9334 (272.8129, 125.1243) -> (272.9735, 125.1224) construction
  line L9335 (272.9735, 125.1224) -> (273.1343, 125.1217) construction
  line L9336 (273.1343, 125.1217) -> (273.2953, 125.122) construction
  line L9337 (273.2953, 125.122) -> (273.4565, 125.1234) construction
  line L9338 (273.4565, 125.1234) -> (273.6179, 125.1258) construction
  line L9339 (273.6179, 125.1258) -> (273.7795, 125.1292) construction
  line L9340 (273.7795, 125.1292) -> (273.9413, 125.1335) construction
  line L9341 (273.9413, 125.1335) -> (274.1032, 125.1389) construction
  line L9342 (274.1032, 125.1389) -> (274.2654, 125.1452) construction
  line L9343 (274.2654, 125.1452) -> (274.4277, 125.1525) construction
  line L9344 (274.4277, 125.1525) -> (274.5901, 125.1608) construction
  line L9345 (274.5901, 125.1608) -> (274.7527, 125.17) construction
  line L9346 (274.7527, 125.17) -> (274.9155, 125.1801) construction
  line L9347 (274.9155, 125.1801) -> (275.0784, 125.1912) construction
  line L9348 (275.0784, 125.1912) -> (275.2415, 125.2033) construction
  line L9349 (275.2415, 125.2033) -> (275.4047, 125.2162) construction
  line L9350 (275.4047, 125.2162) -> (275.568, 125.23) construction
  line L9351 (275.568, 125.23) -> (275.7315, 125.2448) construction
  line L9352 (275.7315, 125.2448) -> (275.8951, 125.2604) construction
  line L9353 (275.8951, 125.2604) -> (276.0588, 125.277) construction
  line L9354 (276.0588, 125.277) -> (276.2226, 125.2944) construction
  line L9355 (276.2226, 125.2944) -> (276.3865, 125.3127) construction
  line L9356 (276.3865, 125.3127) -> (276.5505, 125.3319) construction
  line L9357 (276.5505, 125.3319) -> (276.7146, 125.352) construction
  line L9358 (276.7146, 125.352) -> (276.8788, 125.3729) construction
  line L9359 (276.8788, 125.3729) -> (277.0431, 125.3946) construction
  line L9360 (277.0431, 125.3946) -> (277.2075, 125.4172) construction
  line L9361 (277.2075, 125.4172) -> (277.372, 125.4407) construction
  line L9362 (277.372, 125.4407) -> (277.5366, 125.465) construction
  line L9363 (277.5366, 125.465) -> (277.7012, 125.4902) construction